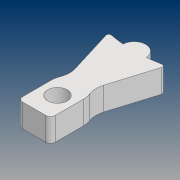
# Autodesk Inventor part: 11_Chot_banh_lai
Saved by Autodesk Inventor 2021 (Build 250183000, 183)
## iProperties
Created: 2024-04-09
Part Number: 11_Chot_banh_lai
Material: Generic
Document SubType Name: Modeling
Designer: Admin
Density: 1 g/cm^3
Appearance: Default
Mass: 1.64712 g
Surface Area: 11.1726 cm^2
Volume: 1.64712 cm^3
Author: Admin
Autodesk Inventor part; units mm, degrees
ref_plane "YZ Plane" through (0, 0, 0) normal (1, 0, 0) x (0, 1, 0)
ref_plane "XZ Plane" through (0, 0, 0) normal (0, 1, 0) x (-1, 0, 0)
ref_plane "XY Plane" through (0, 0, 0) normal (0, 0, 1) x (1, 0, 0)
sketch "Sketch1" plane through (0, 0, 0) normal (0, 1, 0) x (-1, 0, 0)
  line L0 (0, 8.25) -> (0, -8.25) construction
  line L1 (-2.5, 8.25) -> (-2.5, -8.25)
  line L2 (2.5, -8.25) -> (2.5, 8.25)
  arc A0 (2.5, 8.25) -> (-2.5, 8.25) centre (0, 8.25) ccw
  arc A1 (-2.5, -8.25) -> (2.5, -8.25) centre (0, -8.25) ccw
  circle A2 centre (0, 8.25) radius 2.1
  circle A3 centre (0, -8.25) radius 2.1
  line L3 (2.5, 13.25) -> (-2.5, 13.25)
  line L4 (-2.5, 13.25) -> (-2.5, 3.25)
  line L5 (-2.5, 3.25) -> (2.5, 3.25)
  line L6 (2.5, 3.25) -> (2.5, 13.25)
  line L7 (2.5, 13.25) -> (-2.5, 3.25) construction
  line L8 (-2.5, 13.25) -> (2.5, 3.25) construction
  line L9 (0, 8.25) -> (0, -35.75)
  circle A4 centre (0, -35.75) radius 27.5
  line L10 (-6.2348, -8.9661) -> (-2.5, 3.25)
  line L11 (2.5, 3.25) -> (6.2348, -8.9661)
  line L12 (3.5, 13.25) -> (-3.5, 13.25)
  line L13 (-3.5, 13.25) -> (-3.5, 3.25)
  line L14 (-3.5, 3.25) -> (3.5, 3.25)
  line L15 (3.5, 3.25) -> (3.5, 13.25)
  line L16 (3.5, 13.25) -> (-3.5, 3.25) construction
  line L17 (-3.5, 13.25) -> (3.5, 3.25) construction
  point P0 (0, 0)
  point P1 (-2.5, 8.25)
  point P2 (2.5, 8.25)
  point P3 (2.5, 3.25)
  point P4 (2.4974, -8.3636)
  point P5 (-2.4974, -8.3636)
  point P6 (2.5, 3.25)
  point P7 (-2.5, 3.25)
  point P8 (-2.5, 13.25)
  dimension "d1" = 2.5
  dimension "d2" = 4.2
  dimension "d6" = 10
  dimension "d7" = 16.5
  dimension "d8" = 44
  dimension "d9" = 17
  dimension "d12" = 10
  dimension "d13" = 7
  constraints: 38 end point, 7 point on circle, 5 centre point, 5 midpoint, 5 parallel, 4 tangent, 3 coincident, 2 horizontal, 2 perpendicular, 2 vertical, 1 equal radius, 1 point on line, 1 other
  measures "d1" radius of A1
  measures "d2" diameter of A3
  measures "d6" distance between parallel lines of L3 L5
  measures "d7" distance of L9.start A3.centre
  measures "d8" distance of L9.start L9.end
  measures "d9" angle of L1 L10
  measures "d12" distance of L12.end L13.end
  measures "d13" distance between parallel lines of L15 L13
extrude "Extrusion1" add sketch "Sketch1" along normal blind 5 contours A0 L2 L5 L1 | L4 L3 L6 A0 | L1 L14 L13 L12 L4 | L5 L9 A3 A4 A1 L1 | L1 A1 A4 L10 | L6 L12 L15 L14 L2 | L5 L2 A1 A4 A3 L9 | L11 A4 A1 L2 | A4 A3 L9 A1 | L9 A4 A3 | A3 A4 L9 | L9 A3 A4 A1 | A4 L9 A3 | A4 A3 L9
fillet "Fillet2" radius 0.5 2 edges at (6.2348, 2.5, -8.9661) (-6.2348, 2.5, -8.9661)
fillet "Fillet4" radius 4.75 4 edges at (3.5, 2.5, 3.25) (2.5, 2.5, 3.25) (-3.5, 2.5, 3.25) (-2.5, 2.5, 3.25)
fillet "Fillet5" radius 1 2 edges at (-3.5, 2.5, 13.25) (3.5, 2.5, 13.25)
equation "\"d12\" = d6"
body "Solid1"
